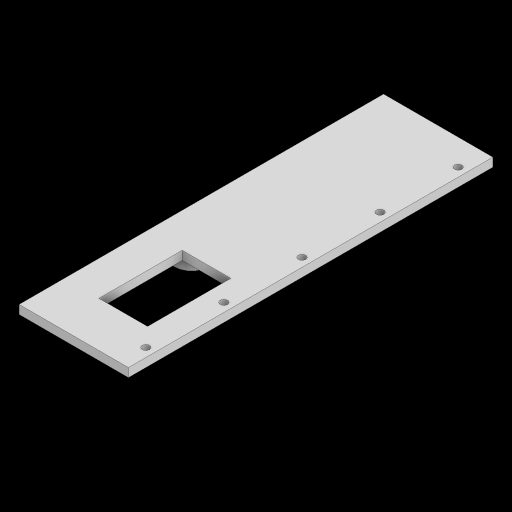
# Autodesk Inventor part: podstawa_sciana_tyl
Saved by Autodesk Inventor 2024.3 (Build 283343000, 343)
## iProperties
Created: 2025-10-10
Part Number: podstawa_sciana_tyl
Material: Ogólny
Document SubType Name: Modeling
Designer: User
Density: 1 g/cm^3
Appearance: Domyślna
Author: User
Autodesk Inventor part; units mm, degrees
ref_plane "YZ Plane" through (0, 0, 0) normal (1, 0, 0) x (0, 1, 0)
sketch "Szkic1" plane through (0, 0, 0) normal (0, 1, 0) x (-1, 0, 0)
  line L0 (-35, 105) -> (35, 105)
  line L1 (35, 105) -> (35, -105)
  line L2 (35, -105) -> (-35, -105)
  line L3 (-35, -105) -> (-35, 105)
  line L4 (-35, 105) -> (35, -105) construction
  line L5 (35, 105) -> (-35, -105) construction
  line L6 (-35, 105) -> (-25, 105)
  line L7 (-30, 105) -> (-30, 90)
  line L8 (35, 105) -> (28, 105)
  line L9 (28, 105) -> (28, -105)
  line L10 (35, -105) -> (28, -105)
  circle A0 centre (-30, 90) radius 2.15
  circle A1 centre (-30, 45) radius 2.15
  circle A2 centre (-30, 0) radius 2.15
  circle A3 centre (-30, -45) radius 2.15
  circle A4 centre (-30, -90) radius 2.15
  line L11 (-35, 105) -> (-35, 55)
  line L12 (-35, 55) -> (-6, 55)
  line L13 (-20, 79) -> (8, 79)
  line L14 (8, 79) -> (8, 31)
  line L15 (8, 31) -> (-20, 31)
  line L16 (-20, 31) -> (-20, 79)
  line L17 (-20, 79) -> (8, 31) construction
  line L18 (8, 79) -> (-20, 31) construction
  point P0 (0, 0)
  point P1 (0, 0)
  dimension "d4" = 70
  dimension "d5" = 210
  dimension "d6" = 10
  dimension "d7" = 15
  dimension "d8" = 7
  dimension "d9" = 4.3
  dimension "d10" = 45
  dimension "d12" = 50
  dimension "d13" = 29
  dimension "d14" = 28
  dimension "d15" = 48
  constraints: 38 end point, 5 centre point, 5 midpoint, 4 parallel, 4 perpendicular, 4 point on line, 3 horizontal, 2 vertical, 1 coincident, 8 other
  measures "d4" distance of L1.end L2.end
  measures "d5" distance of L0.end L1.end
  measures "d6" distance of L0.start L6.end
  measures "d7" distance of L7.start L7.end
  measures "d8" distance of L0.end L8.end
  measures "d9" diameter of A0
  measures "d10" distance of A0.centre A1.centre
  measures "d12" distance of L0.start L11.end
  measures "d13" distance of L11.end L12.end
  measures "d14" distance of L14.end L15.end
  measures "d15" distance of L13.end L14.end
extrude "Wyciągnięcie proste1" add sketch "Szkic1" along normal mid plane 5 contours L0 L9 L2 L3
ref_plane "Płaszczyzna konstrukcyjna1" through (30, -2.5, -105) normal (1, 0, 0) x (0, 0, -1)
ref_plane "Płaszczyzna konstrukcyjna2" through (-23, -2.5, 105) normal (-1, 0, 0) x (0, 0, 1)
sketch "Szkic3" plane through (-23, -2.5, 105) normal (-1, 0, 0) x (0, 0, 1)
  line L0 (-224.7917, 43.2301) -> (-14.7917, 43.2301)
  line L1 (-224.7917, 43.2301) -> (-14.7917, 43.2301)
  line L2 (-119.7917, 43.2301) -> (-119.7917, 58.2301)
  circle A0 centre (-119.7917, 58.2301) radius 2.15
  line L3 (-119.7917, 60.3801) -> (-119.7917, 63.3801)
  line L4 (-150.7917, 43.2301) -> (-198.7917, 43.2301)
  arc A1 (-119.7917, 63.3801) -> (-154.3457, 43.2301) centre (-119.6183, 23.3805) ccw
  arc A2 (-85.2378, 43.2301) -> (-119.7917, 63.3801) centre (-119.9652, 23.3805) ccw
  line L5 (-154.3457, 43.2301) -> (-85.2378, 43.2301)
  line L6 (-210, 0) -> (-210, 5) projected
  line L7 (-210, 0) -> (0, 0) projected
  line L8 (-210, 0) -> (0, 0)
  line L9 (-105, 0) -> (-105, -15)
  circle A3 centre (-105, -15) radius 2.15
  line L10 (-105, -17.15) -> (-105, -20.15)
  arc A4 (-139.554, 0) -> (-105, -20.15) centre (-104.8266, 19.8496) ccw
  arc A5 (-105, -20.15) -> (-70.446, 0) centre (-105.1734, 19.8496) ccw
  line L11 (-70.446, 0) -> (-139.554, 0)
  point P0 (-105, 2.5)
  point P1 (-119.7917, 40.7301)
  point P2 (-70.446, 0)
  point P3 (-139.554, 0)
  dimension "d26" = 4.3
  dimension "d31" = 4.3
  dimension "d25" = 15
  dimension "d27" = 3
  dimension "d28" = 40
  dimension "d29" = 40
  dimension "d30" = 15
  dimension "d32" = 3
  dimension "d33" = 40
  dimension "d34" = 40
  constraints: 20 end point, 8 point on circle, 4 centre point, 4 symmetric about line, 4 vertical, 3 collinear, 2 coincident, 2 midpoint, 2 point on line, 2 vertical alignment, 6 other
  measures "d25" distance of L2.start L2.end
  measures "d27" distance of L3.start L3.end
  measures "d28" distance of L3.end L5.start
  measures "d29" radius of A1
  measures "d30" distance of L9.start L9.end
  measures "d32" distance of L10.start L10.end
  measures "d33" distance of L10.end L11.end
  measures "d34" radius of A4
extrude "Wyciągnięcie proste2" add sketch "Szkic3" against normal blind 7 contours L7 L9 A3 L10 A4 | L7 A5 L10 A3 L9
